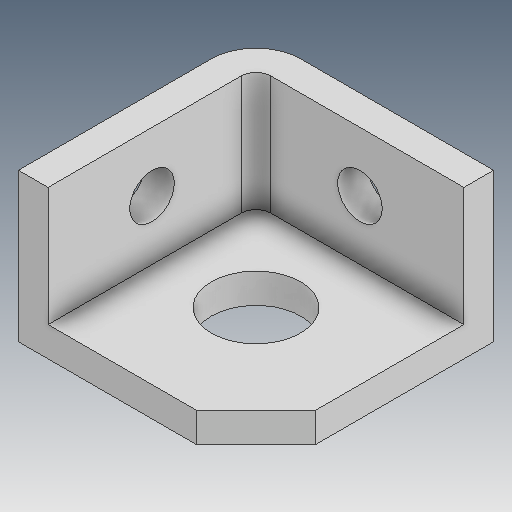
# Autodesk Inventor part: 零件1
Saved by Autodesk Inventor 2025 (Build 290162000, 162)
## iProperties
Created: 2025-03-01
Part Number: 零件1
Material: 常规
Document SubType Name: Modeling
Designer: liukan
Density: 1 g/cm^3
Appearance: 默认
Author: liukan
Autodesk Inventor part; units mm, degrees
ref_plane "YZ Plane" through (0, 0, 0) normal (1, 0, 0) x (0, 1, 0)
ref_plane "XZ Plane" through (0, 0, 0) normal (0, 1, 0) x (-1, 0, 0)
ref_plane "XY Plane" through (0, 0, 0) normal (0, 0, 1) x (1, 0, 0)
sketch "草图1" plane through (0, 0, 0) normal (0, 0, 1) x (1, 0, 0)
  line L0 (0, 0) -> (18, 0) construction
  constraints: 2 end point, 1 horizontal
sketch "草图2" plane through (0, 0, 0) normal (0, 1, 0) x (-1, 0, 0)
  line L0 (40, 40) -> (-40, 40)
  line L1 (-40, 40) -> (-40, -40)
  line L2 (-40, -40) -> (40, -40)
  line L3 (40, -40) -> (40, 40)
  line L4 (40, 40) -> (-40, -40) construction
  line L5 (-40, 40) -> (40, -40) construction
  circle A0 centre (0, 0) radius 15
  line L6 (-20, 40) -> (-40, 20)
  dimension "d4" = 80
  dimension "d5" = 80
  dimension "d6" = 30
  dimension "d7" = 20
  dimension "d8" = 20
  constraints: 14 end point, 2 midpoint, 2 parallel, 2 point on line, 1 centre point, 1 coincident, 1 horizontal, 1 perpendicular
  measures "d4" distance of L2.end L0.start
  measures "d5" distance of L0.start L0.end
  measures "d6" diameter of A0
  measures "d7" distance of L6.end L0.end
  measures "d8" distance of L0.end L6.start
extrude "拉伸1" add sketch "草图2" along normal blind 10 contours L3 L2 L1 L6 L0
sketch "草图3" plane through (0, 10, 0) normal (0, 1, 0) x (1, 0, 0)
  line L0 (40, 40) -> (-40, 40) projected
  line L1 (40, -20) -> (40, 40) projected
  line L2 (-40, 40) -> (40, 40)
  line L3 (40, 40) -> (40, 30)
  line L4 (40, 30) -> (-40, 30)
  line L5 (-40, 30) -> (-40, 40)
  line L6 (-40, -40) -> (20, -40) projected
  line L7 (-40, -40) -> (-30, -40)
  line L8 (-30, -40) -> (-30, 40)
  line L9 (-30, 40) -> (-40, 40)
  line L10 (-40, 40) -> (-40, -40)
  point P0 (0, 0)
  point P1 (-40, 30)
  point P2 (-30, 30)
  dimension "d11" = 10
  dimension "d12" = 10
  constraints: 16 end point, 4 parallel, 2 horizontal, 2 perpendicular, 2 point on line
  measures "d11" distance between parallel lines of L4 L0
  measures "d12" distance between parallel lines of L8 L10
extrude "拉伸2" add sketch "草图3" along normal blind 40
fillet "圆角1" radius 5 1 edges at (-30, 30, -30)
fillet "圆角2" radius 15 1 edges at (-40, 25, -40)
sketch "草图4" plane through (40, 10, -30) normal (0, 0, 1) x (1, 0, 0)
  circle A0 centre (-35, 20) radius 7.5
  line L0 (-65, 40) -> (0, 40) projected
  line L1 (0, 0) -> (0, 40) projected
  point P0 (-40, -10)
  dimension "d17" = 15
  dimension "d18" = 20
  dimension "d19" = 35
  constraints: 1 centre point
  measures "d17" diameter of A0
  measures "d18" distance from line of L0 A0.centre
  measures "d19" distance from line of L1 A0.centre
extrude "拉伸3" cut sketch "草图4" against normal up to next
sketch "草图5" plane through (-30, 10, 40) normal (1, 0, 0) x (0, 0, -1)
  circle A0 centre (35, 20) radius 7.5
  line L0 (0, 0) -> (0, 40) projected
  line L1 (0, 40) -> (65, 40) projected
  point P0 (40, -10)
  dimension "d22" = 15
  dimension "d23" = 35
  dimension "d24" = 20
  constraints: 1 centre point
  measures "d22" diameter of A0
  measures "d23" distance from line of L0 A0.centre
  measures "d24" distance from line of L1 A0.centre
extrude "拉伸4" cut sketch "草图5" against normal up to next
